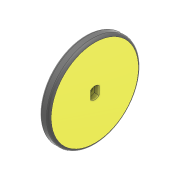
# Autodesk Inventor part: front wheel
Saved by Autodesk Inventor 2022 (Build 260153000, 153)
## iProperties
Created: 2024-04-25
Part Number: front wheel
Material: Generic
Document SubType Name: Modeling
Designer: david
Density: 1 g/cm^3
Appearance: Default
Author: david
Autodesk Inventor part; units mm, degrees
ref_plane "YZ Plane" through (0, 0, 0) normal (1, 0, 0) x (0, 1, 0)
ref_plane "XZ Plane" through (0, 0, 0) normal (0, 1, 0) x (-1, 0, 0)
ref_plane "XY Plane" through (0, 0, 0) normal (0, 0, 1) x (1, 0, 0)
sketch "Sketch1" plane through (0, 0, 0) normal (1, 0, 0) x (0, 1, 0)
  circle A0 centre (0, 0) radius 19
  dimension "d3" = 38
  constraints: 1 centre point, 1 coincident
  measures "d3" diameter of A0
extrude "Extrusion1" add sketch "Sketch1" along normal blind 4
sketch "Sketch2" plane through (4, 0, 0) normal (1, 0, 0) x (0, 0, -1)
  circle A0 centre (0, 0) radius 2.5
  line L0 (-1.75, 1.7854) -> (1.75, 1.7854)
  line L1 (1.75, 1.7854) -> (1.75, -1.7854)
  line L2 (1.75, -1.7854) -> (-1.75, -1.7854)
  line L3 (-1.75, -1.7854) -> (-1.75, 1.7854)
  line L4 (-1.75, 1.7854) -> (1.75, -1.7854) construction
  line L5 (1.75, 1.7854) -> (-1.75, -1.7854) construction
  dimension "d6" = 5
  dimension "d5" = 3.5
  constraints: 12 end point, 2 midpoint, 2 parallel, 1 coincident, 1 horizontal, 1 perpendicular, 3 other
  measures "d5" distance of L1.end L2.end
extrude "Extrusion2" cut sketch "Sketch2" against normal blind 2 contours L0 A0 | L1 L2 L3 L0 | A0 L2
sketch "Sketch3" plane through (2, 0, 0) normal (1, 0, 0) x (0, 0, -1)
  arc A0 (1.75, 1.7854) -> (-1.75, 1.7854) centre (0, 0) ccw projected
  constraints: 1 coincident
hole "Hole1" at (2, 0, 0) direction (-1, 0, 0) diameter 2 end through all
fillet "Fillet1" radius 1 2 edges at (4, -19, 0) (0, -19, 0)
body "Solid1"
